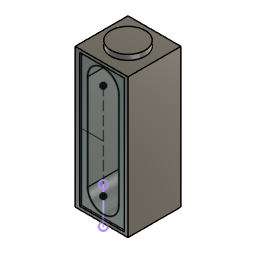
Blaise MagDensitySeperator v10 (Autodesk Fusion 360 archive; units mm, degrees)
design "flow cell"
Autodesk Fusion 360 part; units mm, degrees
sketch "Sketch1" plane through (0, 0, 0) normal (0, 0, 1) x (1, 0, 0) in component "flow cell"
  circle A0 centre (0, 0) radius 9.875
  dimension "d1" = 19.75
  constraint coincident A0.centre origin
  measures "d1" diameter of A0
extrude "Extrude1" add sketch "Sketch1" along normal blind 4.3 in component "flow cell"
sketch "Sketch2" plane through (0, 0, 4.3) normal (0, 0, 1) x (-1, 0, 0) in component "flow cell"
  circle A0 centre (0, 0) radius 9.875
  line L0 (12.7, 12.7) -> (-12.7, 12.7)
  line L1 (-12.7, 12.7) -> (-12.7, -12.7)
  line L2 (-12.7, -12.7) -> (12.7, -12.7)
  line L3 (12.7, -12.7) -> (12.7, 12.7)
  line L4 (12.7, 12.7) -> (-12.7, -12.7) construction
  line L5 (-12.7, 12.7) -> (12.7, -12.7) construction
  line L6 (13.7, 13.7) -> (-13.7, 13.7)
  line L7 (-13.7, 13.7) -> (-13.7, -13.7)
  line L8 (-13.7, -13.7) -> (13.7, -13.7)
  line L9 (13.7, -13.7) -> (13.7, 13.7)
  line L10 (15.2, 15.2) -> (-15.2, 15.2)
  line L11 (-15.2, 15.2) -> (-15.2, -15.2)
  line L12 (-15.2, -15.2) -> (15.2, -15.2)
  line L13 (15.2, -15.2) -> (15.2, 15.2)
  dimension "d4" = 25.4
  dimension "d5" = 25.4
  dimension "d6" = 1
  dimension "d7" = 2.5
  constraint horizontal L0
  constraint perpendicular L0 L1
  constraint parallel L0 L2
  constraint parallel L1 L3
  constraint coincident L4 A0.centre
  constraint coincident L5 A0.centre
  constraint coincident A0.centre origin
  measures "d4" distance of L1.end L2.end
  measures "d5" distance of L0.end L1.end
extrude "Extrude2" add sketch "Sketch2" along normal blind 80 contours A0 | L0 L1 L2 L3 | L6 L7 L8 L9 | L10 L11 L12 L13 in component "flow cell"
sketch "Sketch3" plane through (0, 0, 84.3) normal (0, 0, 1) x (-1, 0, 0) in component "flow cell"
  line L0 (15.2, -15.2) -> (15.2, 15.2)
  line L1 (15.2, 15.2) -> (-15.2, 15.2)
  line L2 (-15.2, 15.2) -> (-15.2, -15.2)
  line L3 (-15.2, -15.2) -> (15.2, -15.2)
  circle A0 centre (0, 0) radius 9.875
  dimension "d10" = 19.75
  constraint coincident A0.centre origin
  measures "d10" diameter of A0
extrude "Extrude3" add sketch "Sketch3" along normal blind 3 contours A0 in component "flow cell"
sketch "Sketch4" plane through (0, -15.2, 0) normal (0, -1, 0) x (1, 0, 0) in component "flow cell"
  line L0 (-15.2, 4.3) -> (15.2, 4.3)
  line L1 (15.2, 4.3) -> (15.2, 84.3)
  line L2 (15.2, 84.3) -> (-15.2, 84.3)
  line L3 (-15.2, 84.3) -> (-15.2, 4.3)
  line L4 (13.0604, 6) -> (-12.5396, 6)
  line L5 (-12.5396, 6) -> (-12.5396, 82.6)
  line L6 (-12.5396, 82.6) -> (13.0604, 82.6)
  line L7 (13.0604, 82.6) -> (13.0604, 6)
  line L8 (13.0604, 6) -> (-12.5396, 82.6) construction
  line L9 (-12.5396, 6) -> (13.0604, 82.6) construction
  line L10 (0.2604, 44.3) -> (-15.2, 44.3) construction
  point P0 (0.2604, 44.3)
  dimension "d13" = 25.6
  dimension "d14" = 76.6
  constraint horizontal L4
  constraint perpendicular L4 L5
  constraint parallel L4 L6
  constraint parallel L5 L7
  constraint coincident L8 P0
  constraint coincident L9 P0
  constraint coincident P0 L10.start
  constraint midpoint L3 L10.end
  constraint horizontal L10
  measures "d13" distance of L5.end L6.end
  measures "d14" distance of L4.end L5.end
extrude "Extrude4" cut sketch "Sketch4" against normal blind 1 contours L4 L5 L6 L7 in component "flow cell"
ref_plane "WorkPlane1" through (0, 0, 44.3) normal (0, -1, 0) x (1, 0, 0) in component "flow cell"
mirror "Mirror1" about plane through (0, 0, 44.3) normal (0, -1, 0) of "Extrude4" in component "flow cell"
sketch "Sketch5" plane through (0, -14.2, 0) normal (0, -1, 0) x (1, 0, 0) in component "flow cell"
  line L0 (13.0604, 82.6) -> (-12.5396, 82.6)
  line L1 (-12.5396, 82.6) -> (-12.5396, 6)
  line L2 (-12.5396, 6) -> (13.0604, 6)
  line L3 (13.0604, 6) -> (13.0604, 82.6)
  line L4 (-9, 71.8) -> (-9, 16.8)
  arc A0 (-9, 16.8) -> (9, 16.8) centre (0, 16.8) ccw
  line L5 (9, 16.8) -> (9, 71.8)
  arc A1 (9, 71.8) -> (-9, 71.8) centre (0, 71.8) ccw
  line L6 (0, 71.8) -> (0, 16.8) construction
  line L7 (-12.5396, 44.3) -> (0, 44.3)
  line L8 (0, 1.75) -> (0, 22.5)
  dimension "d19" = 55
  dimension "d20" = 18
  constraint tangent L4 A0
  constraint tangent A0 L5
  constraint parallel L4 L5
  constraint tangent L5 A1
  constraint tangent L4 A1
  constraint parallel L1 L6
  constraint midpoint L1 L7.start
  constraint midpoint L6 L7.end
  constraint horizontal L7
  constraint collinear L6 L8
  measures "d19" distance of A1.centre A0.centre
  measures "d20" distance of L4 L5
extrude "Extrude5" cut sketch "Sketch5" against normal through all contours L4 A0 L5 A1 in component "flow cell"
component "flow cell" placed x (1, 0, 0) y (0, 1, 0) z (0, 0, 1) at (0, 0, 0)
